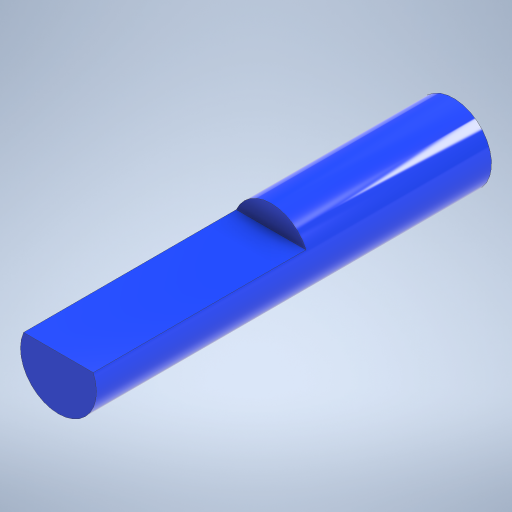
# Autodesk Inventor part: eje steper
Saved by Autodesk Inventor 2023.2 (Build 272271030, 271C)
## iProperties
Created: 2023-03-04
Part Number: eje steper
Material: Generic
Document SubType Name: Modeling
Designer: Cris Pat
Density: 1 g/cm^3
Appearance: Default
Author: Cris Pat
Autodesk Inventor part; units mm, degrees
ref_plane "YZ Plane" through (0, 0, 0) normal (1, 0, 0) x (0, 1, 0)
ref_plane "XZ Plane" through (0, 0, 0) normal (0, 1, 0) x (-1, 0, 0)
ref_plane "XY Plane" through (0, 0, 0) normal (0, 0, 1) x (1, 0, 0)
sketch "Sketch1" plane through (0, 0, 0) normal (0, 0, 1) x (1, 0, 0)
  circle A0 centre (0, 0) radius 2.5
  line L0 (-2.2913, 1) -> (2.2913, 1)
  dimension "d0" = 5
  dimension "d1" = 1
  constraints: 2 end point, 2 point on circle, 1 centre point, 1 coincident, 1 horizontal
  measures "d0" diameter of A0
  measures "d1" distance from line of point (0, 0) L0
extrude "Extrusion1" add sketch "Sketch1" along normal blind 26 contours A0 L0 picked at (0.9904, -1.0234)
extrude "Extrusion2" add sketch "Sketch1" along normal blind 12 contours L0 A0 picked at (0.6667, 1.1666)
body "Solid1"
